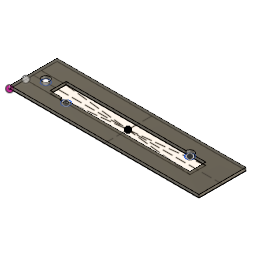
lan switch plate (Autodesk Fusion 360 design; units mm, degrees)
Autodesk Fusion 360 part; units mm, degrees
sketch "Sketch1" plane through (0, 0, 0) normal (0, 0, 1) x (1, 0, 0)
  line L0 (0, 0) -> (609.6, 0)
  line L1 (609.6, 0) -> (609.6, 152.4)
  line L2 (609.6, 152.4) -> (0, 152.4)
  line L3 (0, 152.4) -> (0, 0)
  line L4 (0, 0) -> (0, 53.848)
  line L5 (0, 76.2) -> (609.6, 76.2) construction
  line L6 (304.8, 152.4) -> (304.8, 0) construction
  line L7 (529.8, 101.6) -> (79.8, 101.6)
  line L8 (79.8, 101.6) -> (79.8, 50.8)
  line L9 (79.8, 50.8) -> (529.8, 50.8)
  line L10 (529.8, 50.8) -> (529.8, 101.6)
  line L11 (529.8, 101.6) -> (79.8, 50.8) construction
  line L12 (79.8, 101.6) -> (529.8, 50.8) construction
  line L13 (79.8, 101.6) -> (0, 101.6)
  line L14 (79.8, 50.8) -> (0, 50.8)
  circle A0 centre (39.9, 76.2) radius 12.7
  line L15 (79.8, 50.8) -> (130.6, 50.8)
  circle A1 centre (130.6, 50.8) radius 12.7
  line L16 (529.8, 101.6) -> (508, 101.6)
  line L17 (529.8, 101.6) -> (479, 101.6)
  circle A2 centre (479, 101.6) radius 12.7
  point P0 (304.8, 76.2)
  dimension "d1" = 609.6
  dimension "d2" = 152.4
  dimension "d12" = 450
  dimension "d13" = 50.8
  dimension "d14" = 25.4
  dimension "d16" = 25.4
  dimension "d18" = 25.4
  constraint horizontal L0
  constraint vertical L1
  constraint horizontal L2
  constraint vertical L3
  constraint coincident L0.start L3.end
  constraint perpendicular L0 L4
  constraint midpoint L3 L5.start
  constraint midpoint L1 L5.end
  constraint midpoint L2 L6.start
  constraint midpoint L0 L6.end
  constraint perpendicular L7 L8
  constraint parallel L7 L9
  constraint parallel L8 L10
  constraint horizontal L7
  constraint coincident L11 P0
  constraint coincident L12 P0
  constraint midpoint L6 P0
  constraint coincident L3 L13.end
  constraint perpendicular L3 L13
  constraint perpendicular L8 L14
  constraint perpendicular L8 L15
  constraint coincident L15.end A1.centre
  constraint coincident L7 L16.end
  constraint perpendicular L10 L17
  constraint coincident L17.end A2.centre
  measures "d1" distance of L0.start L0.end
  measures "d2" distance of L0.start L2.end
  measures "d12" distance of L8.end L9.end
  measures "d13" distance of L7.end L8.end
  measures "d14" diameter of A0
  measures "d16" diameter of A1
  measures "d18" diameter of A2
extrude "Extrude1" add sketch "Sketch1" along normal blind 9.525 contours L0 L1 L2 L3 L4 L7 L9 L10 L13 L14 L15 A1 L16 L17 A2 | L3 L4 L8 L13 L14
equation "d1 = 2'-0\""
equation "d2 = 6\""
equation "d8 = ( 3 / 8 ) * 1 in"
equation "d14 = 1\""
equation "d16 = 1\""
equation "d18 = 1\""
